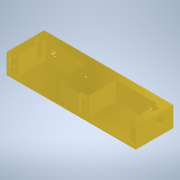
# Autodesk Inventor part: Part4
Saved by Autodesk Inventor 2022 (Build 260153000, 153)
## iProperties
Created: 2021-06-22
Part Number: Part4
Material: Generic
Document SubType Name: Modeling
Designer: Prajwal Patil
Density: 1 g/cm^3
Appearance: Diamond Plate
Author: Prajwal Patil
Autodesk Inventor part; units mm, degrees
ref_plane "YZ Plane" through (0, 0, 0) normal (1, 0, 0) x (0, 1, 0)
ref_plane "XZ Plane" through (0, 0, 0) normal (0, 1, 0) x (-1, 0, 0)
ref_plane "XY Plane" through (0, 0, 0) normal (0, 0, 1) x (1, 0, 0)
sketch "Sketch2" plane through (0, 0, 0) normal (0, 1, 0) x (-1, 0, 0)
  line L0 (77.2994, 22.4824) -> (-85.2606, 22.4824)
  line L1 (-85.2606, 22.4824) -> (-85.2606, -24.5076)
  line L2 (-85.2606, -24.5076) -> (77.2994, -24.5076)
  line L3 (77.2994, -24.5076) -> (77.2994, 22.4824)
  point P0 (0, 0)
  dimension "d0" = 162.56
  dimension "d1" = 46.99
  constraints: 8 end point, 2 parallel, 1 horizontal, 1 perpendicular
  measures "d0" distance of L2.end L1.end
  measures "d1" distance of L1.end L0.end
extrude "Extrusion1" add sketch "Sketch2" along normal blind 25.4
sketch "Sketch3" plane through (0, 25.4, 0) normal (0, 1, 0) x (1, 0, 0)
  point P0 (0, 0)
sketch "Sketch4" plane through (0, 25.4, 0) normal (0, 1, 0) x (1, 0, 0)
  line L0 (85.2606, -22.4824) -> (85.2606, 24.5076) projected
  line L1 (74.5926, -22.4824) -> (74.5926, 15.6176)
  line L2 (74.5926, 15.6176) -> (22.2686, 15.6176)
  line L3 (22.2686, 15.6176) -> (22.2686, -22.4824)
  line L4 (-14.3074, -22.4824) -> (-14.3074, 15.6176)
  line L5 (-14.3074, 15.6176) -> (-66.6314, 15.6176)
  line L6 (-66.6314, 15.6176) -> (-66.6314, -22.4824)
  line L7 (-66.6314, -22.4824) -> (-14.3074, -22.4824)
  line L8 (22.2686, -22.4824) -> (74.5926, -22.4824)
  point P0 (0, 0)
  dimension "d4" = 10.668
  dimension "d5" = 38.1
  dimension "d6" = 52.324
  dimension "d7" = 36.576
  dimension "d8" = 52.324
  constraints: 16 end point, 3 perpendicular, 1 collinear
  measures "d4" distance of L0.start L1.start
  measures "d5" distance of L1.start L1.end
  measures "d6" distance of L1.end L2.end
  measures "d7" distance of L3.end L4.start
  measures "d8" distance of L4.end L5.end
extrude "Extrusion2" cut sketch "Sketch4" against normal blind 23.495
sketch "Sketch5" plane through (0, 25.4, 0) normal (0, 1, 0) x (1, 0, 0)
  line L0 (74.5926, -22.4824) -> (22.2686, -22.4824) projected
  line L1 (22.2686, -22.4824) -> (13.5564, -22.4824)
  line L2 (13.5564, -22.4824) -> (13.5564, -18.6724)
  line L3 (13.5564, -18.6724) -> (22.2686, -18.6724)
  line L4 (22.2686, -18.6724) -> (22.2686, -22.4824)
  line L5 (-14.3074, -22.4824) -> (22.2686, -22.4824) projected
  line L6 (-14.3074, -22.4824) -> (-5.5952, -22.4824)
  line L7 (-5.5952, -22.4824) -> (-5.5952, -18.6724)
  line L8 (-5.5952, -18.6724) -> (-14.3074, -18.6724)
  line L9 (-14.3074, -18.6724) -> (-14.3074, -22.4824)
  line L10 (74.5926, -22.4824) -> (85.2606, -22.4824) projected
  line L11 (74.5926, -22.4824) -> (83.3048, -22.4824)
  line L12 (83.3048, -22.4824) -> (83.3048, -18.6724)
  line L13 (83.3048, -18.6724) -> (74.5926, -18.6724)
  line L14 (74.5926, -18.6724) -> (74.5926, -22.4824)
  line L15 (-66.6314, -22.4824) -> (-66.6314, 15.6176) projected
  line L16 (-66.6314, -22.4824) -> (-75.3436, -22.4824)
  line L17 (-75.3436, -22.4824) -> (-75.3436, -18.6724)
  line L18 (-75.3436, -18.6724) -> (-66.6314, -18.6724)
  line L19 (-66.6314, -18.6724) -> (-66.6314, -22.4824)
  point P0 (0, 0)
  point P1 (-77.2994, -22.4824)
  dimension "d11" = 8.7122
  dimension "d12" = 3.81
  dimension "d13" = 8.7122
  dimension "d14" = 3.81
  dimension "d18" = 8.7122
  dimension "d19" = 8.7122
  dimension "d20" = 3.81
  constraints: 32 end point, 8 parallel, 4 horizontal, 4 perpendicular
  measures "d11" distance of L2.end L3.end
  measures "d12" distance of L1.end L2.end
  measures "d13" distance of L8.end L7.end
  measures "d14" distance of L7.end L6.end
  measures "d18" distance of L13.end L12.end
  measures "d19" distance of L17.end L18.end
  measures "d20" distance of L16.end L17.end
extrude "Extrusion3" cut sketch "Sketch5" against normal blind 22.5552
sketch "Sketch6" plane through (0, 25.4, 0) normal (0, 1, 0) x (1, 0, 0)
  line L0 (74.5926, 12.4426) -> (79.7234, 12.4426)
  line L1 (79.7234, 12.4426) -> (79.7234, 4.8226)
  line L2 (79.7234, 4.8226) -> (74.5926, 4.8226)
  line L3 (74.5926, 12.4426) -> (74.5926, 4.8226)
  line L4 (-66.6314, 12.4426) -> (-71.7622, 12.4426)
  line L5 (-71.7622, 12.4426) -> (-71.7622, 4.8226)
  line L6 (-71.7622, 4.8226) -> (-66.6314, 4.8226)
  line L7 (-66.6314, 4.8226) -> (-66.6314, 12.4426)
  point P0 (0, 0)
  point P1 (74.5926, 15.6176)
  point P2 (-66.6314, 15.6176)
  dimension "d23" = 3.175
  dimension "d24" = 5.1308
  dimension "d25" = 7.62
  dimension "d26" = 3.175
  dimension "d27" = 5.1308
  constraints: 16 end point, 3 perpendicular, 2 horizontal, 1 vertical
  measures "d23" distance of point (74.593, 15.618) L0.start
  measures "d24" distance of L0.start L0.end
  measures "d25" distance of L0.end L1.end
  measures "d26" distance of point (-66.631, 15.618) L4.start
  measures "d27" distance of L4.start L4.end
extrude "Extrusion4" cut sketch "Sketch6" against normal blind 15.875
sketch "Sketch7" plane through (85.2606, 0, 22.4824) normal (1, 0, 0) x (0, 0, -1)
  point P0 (22.4824, 0)
sketch "Sketch8" plane through (85.2606, 0, 22.4824) normal (1, 0, 0) x (0, 0, -1)
  line L0 (27.305, 9.525) -> (34.925, 9.525) projected
  line L1 (27.305, 25.4) -> (27.305, 9.525) projected
  line L2 (34.925, 9.525) -> (27.305, 9.525)
  line L3 (27.305, 9.525) -> (27.305, 20.955)
  line L4 (27.305, 20.955) -> (34.925, 20.955)
  line L5 (38.1, 25.4) -> (38.1, 1.905) projected
  line L6 (34.925, 20.955) -> (34.925, 9.525)
  point P0 (22.4824, 0)
  point P1 (46.99, 0)
  dimension "d32" = 11.43
  constraints: 8 end point, 1 perpendicular, 1 point on line
  measures "d32" distance of L0.start L3.end
extrude "Extrusion5" cut sketch "Sketch8" against normal blind 10.3124
sketch "Sketch10" plane through (-77.2994, 0, -24.5076) normal (-1, 0, 0) x (0, 0, 1)
  line L0 (19.685, 20.955) -> (12.065, 20.955) projected
  line L1 (19.685, 9.525) -> (19.685, 20.955) projected
  line L2 (12.065, 20.955) -> (19.685, 20.955)
  line L3 (19.685, 20.955) -> (19.685, 9.525)
  line L4 (19.685, 9.525) -> (12.065, 9.525)
  line L5 (12.065, 9.525) -> (12.065, 20.955)
  point P0 (24.5076, 0)
  constraints: 8 end point, 2 parallel, 1 horizontal, 1 perpendicular
extrude "Extrusion6" cut sketch "Sketch10" against normal blind 10.3124
sketch "Sketch12" plane through (74.5926, 25.4, 18.6724) normal (0, 0, 1) x (1, 0, 0)
  line L0 (8.7122, -22.5552) -> (4.9022, -22.5552)
  line L1 (-61.0362, 0) -> (-61.0362, -22.5552) projected
  line L2 (-61.0362, -22.5552) -> (-57.2262, -22.5552)
  line L3 (-61.0362, -22.5552) -> (-52.324, -22.5552) projected
  line L4 (8.7122, -22.5552) -> (0, -22.5552) projected
  line L5 (8.7122, -22.5552) -> (4.9022, -22.5552)
  line L6 (10.668, -15.875) -> (0, -15.875) projected
  line L7 (4.9022, -22.5552) -> (12.5222, -22.5552) construction
  circle A0 centre (4.9022, -14.9352) radius 1.27
  circle A1 centre (4.9022, -4.1402) radius 1.27
  circle A2 centre (-57.2262, -4.1402) radius 1.27
  circle A3 centre (-57.2262, -14.9352) radius 1.27
  line L8 (-80.1878, -22.5552) -> (-83.9978, -22.5552)
  line L9 (-80.1878, -22.5552) -> (-88.9, -22.5552) projected
  circle A4 centre (-83.9978, -4.1402) radius 1.27
  circle A5 centre (-83.9978, -14.9352) radius 1.27
  line L10 (-141.224, -22.5552) -> (-149.9362, -22.5552) projected
  line L11 (-149.9362, -22.5552) -> (-146.1262, -22.5552)
  line L12 (-146.1262, -14.9352) -> (-135.3312, -14.9352) construction
  circle A6 centre (-146.1262, -14.9352) radius 1.27
  circle A7 centre (-146.1262, -4.1402) radius 1.27
  point P0 (-74.5926, -25.4)
  dimension "d48" = 3.81
  dimension "d55" = 2.54
  dimension "d56" = 2.54
  dimension "d57" = 3.81
  dimension "d58" = 2.54
  dimension "d59" = 2.54
  dimension "d60" = 3.81
  dimension "d64" = 2.54
  dimension "d65" = 2.54
  constraints: 14 end point, 8 centre point, 3 point on line, 2 horizontal, 1 coincident, 1 collinear
  measures "d48" distance of L1.end L2.end
  measures "d55" diameter of A0
  measures "d56" diameter of A1
  measures "d57" distance of L8.start L8.end
  measures "d58" diameter of A4
  measures "d59" diameter of A5
  measures "d60" distance of L10.end L11.end
  measures "d64" diameter of A6
  measures "d65" diameter of A7
extrude "Extrusion7" cut sketch "Sketch12" against normal blind 10.16
sketch "Sketch13" plane through (22.2686, 25.4, -15.6176) normal (0, 0, 1) x (1, 0, 0)
  line L0 (52.324, -23.495) -> (0, -23.495) projected
  line L1 (52.324, -23.495) -> (42.164, -23.495)
  circle A0 centre (42.164, -10.16) radius 3.81
  line L2 (-88.9, -23.495) -> (-36.576, -23.495) projected
  line L3 (-88.9, -23.495) -> (-78.74, -23.495)
  line L4 (62.992, -25.4) -> (-99.568, -25.4) projected
  line L5 (-88.9, -23.495) -> (-78.74, -23.495) construction
  circle A1 centre (-78.74, -10.16) radius 3.81
  point P0 (-22.2686, -25.4)
  dimension "d68" = 10.16
  dimension "d70" = 7.62
  dimension "d71" = 10.16
  dimension "d72" = 0
  dimension "d73" = 7.62
  constraints: 6 end point, 2 centre point, 1 collinear, 1 horizontal, 1 parallel, 1 point on line
  measures "d68" distance of L0.start L1.end
  measures "d70" diameter of A0
  measures "d71" distance of L2.start L3.end
  measures "d72" distance between parallel lines of L3 L5
  measures "d73" diameter of A1
extrude "Extrusion8" cut sketch "Sketch13" against normal blind 8.89
sketch "Sketch14" plane through (0, 0, 0) normal (0, -1, 0) x (1, 0, 0)
  line L0 (-74.5451, 20.5131) -> (78.1896, 20.5131) construction
  line L1 (78.1896, 20.5131) -> (78.1896, -20.8075) construction
  line L2 (78.1896, -20.8075) -> (-74.5451, -20.8075) construction
  line L3 (-74.5451, -20.8075) -> (-74.5451, 20.5131) construction
  spline S0 degree 2 poles (-33.4111, 7.8193) (-33.4111, 6.4937) (-34.4197, 4.4621) (-35.2554, 3.7993) knots 0 0 0 1 2 2 2
  spline S1 degree 2 poles (-35.2554, 3.7993) (-36.264, 3.0213) (-38.5549, 2.3585) (-40.3704, 2.3585) knots 0 0 0 1 2 2 2
  line L4 (-40.3704, 2.3585) -> (-45.471, 2.3585)
  line L5 (-45.471, 2.3585) -> (-45.471, 20.1385)
  line L6 (-45.471, 20.1385) -> (-40.7594, 20.1385)
  spline S2 degree 2 poles (-40.7594, 20.1385) (-38.8575, 20.1385) (-36.9556, 19.8935) (-36.0911, 19.4181) knots 0 0 0 1 2 2 2
  spline S3 degree 2 poles (-36.0911, 19.4181) (-35.1257, 18.9138) (-34.2468, 17.2568) (-34.2468, 16.1329) knots 0 0 0 1 2 2 2
  spline S4 degree 2 poles (-34.2468, 16.1329) (-34.2468, 14.8794) (-35.5724, 12.891) (-36.7394, 12.3291) knots 0 0 0 1 2 2 2
  line L7 (-36.7394, 12.3291) -> (-36.7394, 12.2427)
  spline S5 degree 2 poles (-36.7394, 12.2427) (-35.1545, 11.8104) (-33.4111, 9.5195) (-33.4111, 7.8193) knots 0 0 0 1 2 2 2
  spline S6 degree 2 poles (-35.8749, 7.7184) (-35.8749, 8.727) (-36.4513, 10.0238) (-37.3158, 10.4848) knots 0 0 0 1 2 2 2
  spline S7 degree 2 poles (-37.3158, 10.4848) (-37.8777, 10.773) (-39.2033, 10.9459) (-40.428, 10.9459) knots 0 0 0 1 2 2 2
  line L8 (-40.428, 10.9459) -> (-43.108, 10.9459)
  line L9 (-43.108, 10.9459) -> (-43.108, 4.3757)
  line L10 (-43.108, 4.3757) -> (-41.1917, 4.3757)
  spline S8 degree 2 poles (-41.1917, 4.3757) (-39.6355, 4.3757) (-37.8489, 4.6638) (-37.1573, 5.1249) knots 0 0 0 1 2 2 2
  spline S9 degree 2 poles (-37.1573, 5.1249) (-36.4945, 5.6004) (-35.8749, 6.7819) (-35.8749, 7.7184) knots 0 0 0 1 2 2 2
  spline S10 degree 2 poles (-36.7106, 15.8015) (-36.7106, 16.4355) (-37.1429, 17.3865) (-37.6184, 17.6602) knots 0 0 0 1 2 2 2
  spline S11 degree 2 poles (-37.6184, 17.6602) (-38.1947, 17.9772) (-39.5923, 18.1213) (-40.8459, 18.1213) knots 0 0 0 1 2 2 2
  line L11 (-40.8459, 18.1213) -> (-43.108, 18.1213)
  line L12 (-43.108, 18.1213) -> (-43.108, 12.9199)
  line L13 (-43.108, 12.9199) -> (-40.428, 12.9199)
  spline S12 degree 2 poles (-40.428, 12.9199) (-39.3186, 12.9199) (-38.2667, 13.1504) (-37.7048, 13.5106) knots 0 0 0 1 2 2 2
  spline S13 degree 2 poles (-37.7048, 13.5106) (-37.1573, 13.8564) (-36.7106, 14.9658) (-36.7106, 15.8015) knots 0 0 0 1 2 2 2
  spline S14 degree 2 poles (-18.484, 18.1069) (-17.4754, 16.9254) (-16.3515, 13.4674) (-16.3515, 11.2485) knots 0 0 0 1 2 2 2
  spline S15 degree 2 poles (-16.3515, 11.2485) (-16.3515, 9.0872) (-17.4466, 5.586) (-18.484, 4.4045) knots 0 0 0 1 2 2 2
  spline S16 degree 2 poles (-18.484, 4.4045) (-19.579, 3.1653) (-22.4751, 1.9839) (-24.2185, 1.9839) knots 0 0 0 1 2 2 2
  spline S17 degree 2 poles (-24.2185, 1.9839) (-26.0196, 1.9839) (-28.9013, 3.2086) (-29.9531, 4.4045) knots 0 0 0 1 2 2 2
  spline S18 degree 2 poles (-29.9531, 4.4045) (-30.9761, 5.586) (-32.0711, 9.0584) (-32.0711, 11.2485) knots 0 0 0 1 2 2 2
  spline S19 degree 2 poles (-32.0711, 11.2485) (-32.0711, 13.4818) (-30.9617, 16.8822) (-29.9387, 18.1069) knots 0 0 0 1 2 2 2
  spline S20 degree 2 poles (-29.9387, 18.1069) (-28.9013, 19.2884) (-26.0052, 20.5131) (-24.2185, 20.5131) knots 0 0 0 1 2 2 2
  spline S21 degree 2 poles (-24.2185, 20.5131) (-22.4031, 20.5131) (-19.4926, 19.2452) (-18.484, 18.1069) knots 0 0 0 1 2 2 2
  spline S22 degree 2 poles (-18.8154, 11.2485) (-18.8154, 13.0063) (-19.579, 15.7295) (-20.2706, 16.6228) knots 0 0 0 1 2 2 2
  spline S23 degree 2 poles (-20.2706, 16.6228) (-20.9766, 17.545) (-22.965, 18.4671) (-24.2041, 18.4671) knots 0 0 0 1 2 2 2
  spline S24 degree 2 poles (-24.2041, 18.4671) (-25.4865, 18.4671) (-27.4172, 17.5738) (-28.152, 16.6228) knots 0 0 0 1 2 2 2
  spline S25 degree 2 poles (-28.152, 16.6228) (-28.858, 15.7151) (-29.6073, 12.9775) (-29.6073, 11.2485) knots 0 0 0 1 2 2 2
  spline S26 degree 2 poles (-29.6073, 11.2485) (-29.6073, 7.7472) (-26.668, 4.0299) (-24.2041, 4.0299) knots 0 0 0 1 2 2 2
  spline S27 degree 2 poles (-24.2041, 4.0299) (-21.7403, 4.0299) (-18.8154, 7.7472) (-18.8154, 11.2485) knots 0 0 0 1 2 2 2
  line L14 (-9.6084, 2.3585) -> (-9.6084, 18.0348)
  line L15 (-9.6084, 18.0348) -> (-15.5735, 18.0348)
  line L16 (-15.5735, 18.0348) -> (-15.5735, 20.1385)
  line L17 (-15.5735, 20.1385) -> (-1.2803, 20.1385)
  line L18 (-1.2803, 20.1385) -> (-1.2803, 18.0348)
  line L19 (-1.2803, 18.0348) -> (-7.2454, 18.0348)
  line L20 (-7.2454, 18.0348) -> (-7.2454, 2.3585)
  line L21 (-7.2454, 2.3585) -> (-9.6084, 2.3585)
  line L22 (6.5291, 9.0584) -> (-0.1997, 9.0584)
  line L23 (-0.1997, 9.0584) -> (-0.1997, 11.2197)
  line L24 (-0.1997, 11.2197) -> (6.5291, 11.2197)
  line L25 (6.5291, 11.2197) -> (6.5291, 9.0584)
  line L26 (18.9635, 2.3585) -> (10.2897, 2.3585)
  line L27 (10.2897, 2.3585) -> (10.2897, 4.1739)
  line L28 (10.2897, 4.1739) -> (13.5171, 4.1739)
  line L29 (13.5171, 4.1739) -> (13.5171, 16.0897)
  line L30 (13.5171, 16.0897) -> (10.2897, 16.0897)
  line L31 (10.2897, 16.0897) -> (10.2897, 17.7179)
  spline S28 degree 2 poles (10.2897, 17.7179) (12.1195, 17.7179) (13.8485, 18.7553) (13.9638, 20.1961) knots 0 0 0 1 2 2 2
  line L32 (13.9638, 20.1961) -> (15.8081, 20.1961)
  line L33 (15.8081, 20.1961) -> (15.8081, 4.1739)
  line L34 (15.8081, 4.1739) -> (18.9635, 4.1739)
  line L35 (18.9635, 4.1739) -> (18.9635, 2.3585)
  spline S29 degree 2 poles (33.4728, 8.1218) (33.4728, 6.753) (32.5651, 4.4333) (31.8014, 3.6552) knots 0 0 0 1 2 2 2
  spline S30 degree 2 poles (31.8014, 3.6552) (31.009, 2.834) (29.0206, 1.9839) (27.8247, 1.9839) knots 0 0 0 1 2 2 2
  spline S31 degree 2 poles (27.8247, 1.9839) (26.6288, 1.9839) (24.6549, 2.7907) (23.9056, 3.5976) knots 0 0 0 1 2 2 2
  spline S32 degree 2 poles (23.9056, 3.5976) (22.9835, 4.563) (21.9461, 7.8049) (21.9461, 10.1678) knots 0 0 0 1 2 2 2
  spline S33 degree 2 poles (21.9461, 10.1678) (21.9461, 12.4876) (22.897, 16.2194) (23.8912, 17.6026) knots 0 0 0 1 2 2 2
  spline S34 degree 2 poles (23.8912, 17.6026) (24.8566, 18.957) (27.9112, 20.4699) (29.9139, 20.4699) knots 0 0 0 1 2 2 2
  spline S35 degree 2 poles (29.9139, 20.4699) (30.5047, 20.4699) (31.5421, 20.3546) (31.9311, 20.2249) knots 0 0 0 1 2 2 2
  line L36 (31.9311, 20.2249) -> (31.9311, 17.934)
  line L37 (31.9311, 17.934) -> (31.8303, 17.934)
  spline S36 degree 2 poles (31.8303, 17.934) (31.4989, 18.1069) (30.2886, 18.4095) (29.597, 18.4095) knots 0 0 0 1 2 2 2
  spline S37 degree 2 poles (29.597, 18.4095) (27.3781, 18.4095) (24.6549, 15.4125) (24.3955, 12.4732) knots 0 0 0 1 2 2 2
  spline S38 degree 2 poles (24.3955, 12.4732) (25.2456, 13.0639) (27.0323, 13.7123) (28.0985, 13.7123) knots 0 0 0 1 2 2 2
  spline S39 degree 2 poles (28.0985, 13.7123) (29.1359, 13.7123) (30.692, 13.2945) (31.5421, 12.6605) knots 0 0 0 1 2 2 2
  spline S40 degree 2 poles (31.5421, 12.6605) (32.5219, 11.9257) (33.4728, 9.6491) (33.4728, 8.1218) knots 0 0 0 1 2 2 2
  spline S41 degree 2 poles (31.0522, 8.021) (31.0522, 9.116) (30.4759, 10.6001) (29.8419, 11.1188) knots 0 0 0 1 2 2 2
  spline S42 degree 2 poles (29.8419, 11.1188) (29.3664, 11.4934) (28.1849, 11.7384) (27.5654, 11.7384) knots 0 0 0 1 2 2 2
  spline S43 degree 2 poles (27.5654, 11.7384) (26.7297, 11.7384) (25.1592, 11.2341) (24.3955, 10.7586) knots 0 0 0 1 2 2 2
  spline S44 degree 2 poles (24.3955, 10.7586) (24.3811, 10.4992) (24.3523, 10.0093) (24.3523, 9.6347) knots 0 0 0 1 2 2 2
  spline S45 degree 2 poles (24.3523, 9.6347) (24.3523, 7.7905) (25.0727, 5.5283) (25.6202, 4.9376) knots 0 0 0 1 2 2 2
  spline S46 degree 2 poles (25.6202, 4.9376) (26.1245, 4.3757) (27.2196, 3.929) (27.8391, 3.929) knots 0 0 0 1 2 2 2
  spline S47 degree 2 poles (27.8391, 3.929) (29.28, 3.929) (31.0522, 5.975) (31.0522, 8.021) knots 0 0 0 1 2 2 2
  spline S48 degree 2 poles (-38.1227, -15.5926) (-38.1227, -17.9289) (-40.3868, -20.7797) (-42.0953, -20.7797) knots 0 0 0 1 2 2 2
  spline S49 degree 2 poles (-42.0953, -20.7797) (-42.8671, -20.7797) (-43.9684, -20.3989) (-44.5035, -20.0695) knots 0 0 0 1 2 2 2
  line L38 (-44.5035, -20.0695) -> (-44.6064, -20.5121)
  line L39 (-44.6064, -20.5121) -> (-46.109, -20.5121)
  line L40 (-46.109, -20.5121) -> (-46.109, -7.246)
  line L41 (-46.109, -7.246) -> (-44.5035, -7.246)
  line L42 (-44.5035, -7.246) -> (-44.5035, -11.9802)
  spline S50 degree 2 poles (-44.5035, -11.9802) (-43.8963, -11.4348) (-42.4864, -10.7144) (-41.591, -10.7144) knots 0 0 0 1 2 2 2
  spline S51 degree 2 poles (-41.591, -10.7144) (-39.9752, -10.7144) (-38.1227, -13.2976) (-38.1227, -15.5926) knots 0 0 0 1 2 2 2
  spline S52 degree 2 poles (-39.7796, -15.7161) (-39.7796, -14.0077) (-40.8191, -12.2375) (-41.9718, -12.2375) knots 0 0 0 1 2 2 2
  spline S53 degree 2 poles (-41.9718, -12.2375) (-42.6201, -12.2375) (-43.9581, -12.855) (-44.5035, -13.3285) knots 0 0 0 1 2 2 2
  line L43 (-44.5035, -13.3285) -> (-44.5035, -18.7934)
  spline S54 degree 2 poles (-44.5035, -18.7934) (-43.8963, -19.0918) (-42.9598, -19.3388) (-42.404, -19.3388) knots 0 0 0 1 2 2 2
  spline S55 degree 2 poles (-42.404, -19.3388) (-41.1793, -19.3388) (-39.7796, -17.5995) (-39.7796, -15.7161) knots 0 0 0 1 2 2 2
  line L44 (-28.9733, -10.9819) -> (-34.0986, -24.0216)
  line L45 (-34.0986, -24.0216) -> (-35.8173, -24.0216)
  line L46 (-35.8173, -24.0216) -> (-34.1089, -20.049)
  line L47 (-34.1089, -20.049) -> (-37.5669, -10.9819)
  line L48 (-37.5669, -10.9819) -> (-35.8379, -10.9819)
  line L49 (-35.8379, -10.9819) -> (-33.2341, -18.0421)
  line L50 (-33.2341, -18.0421) -> (-30.6406, -10.9819)
  line L51 (-30.6406, -10.9819) -> (-28.9733, -10.9819)
  line L52 (-19.2167, -20.5121) -> (-19.2167, -9.3147)
  line L53 (-19.2167, -9.3147) -> (-23.4775, -9.3147)
  line L54 (-23.4775, -9.3147) -> (-23.4775, -7.8121)
  line L55 (-23.4775, -7.8121) -> (-13.2681, -7.8121)
  line L56 (-13.2681, -7.8121) -> (-13.2681, -9.3147)
  line L57 (-13.2681, -9.3147) -> (-17.5289, -9.3147)
  line L58 (-17.5289, -9.3147) -> (-17.5289, -20.5121)
  line L59 (-17.5289, -20.5121) -> (-19.2167, -20.5121)
  spline S56 degree 2 poles (-7.9679, -20.7282) (-10.2526, -20.7282) (-12.7638, -18.1656) (-12.7638, -15.7985) knots 0 0 0 1 2 2 2
  spline S57 degree 2 poles (-12.7638, -15.7985) (-12.7638, -13.4725) (-10.3247, -10.7144) (-8.359, -10.7144) knots 0 0 0 1 2 2 2
  spline S58 degree 2 poles (-8.359, -10.7144) (-7.4739, -10.7144) (-6.1051, -11.2289) (-5.6008, -11.7744) knots 0 0 0 1 2 2 2
  spline S59 degree 2 poles (-5.6008, -11.7744) (-5.0862, -12.3199) (-4.5407, -13.8945) (-4.5407, -15.0369) knots 0 0 0 1 2 2 2
  line L60 (-4.5407, -15.0369) -> (-4.5407, -15.9117)
  line L61 (-4.5407, -15.9117) -> (-11.1377, -15.9117)
  spline S60 degree 2 poles (-11.1377, -15.9117) (-11.1377, -17.5686) (-9.4705, -19.3285) (-7.9885, -19.3285) knots 0 0 0 1 2 2 2
  spline S61 degree 2 poles (-7.9885, -19.3285) (-7.4636, -19.3285) (-6.4447, -19.0918) (-6.033, -18.9066) knots 0 0 0 1 2 2 2
  spline S62 degree 2 poles (-6.033, -18.9066) (-5.6008, -18.7007) (-5.0039, -18.3405) (-4.8083, -18.1759) knots 0 0 0 1 2 2 2
  line L62 (-4.8083, -18.1759) -> (-4.7157, -18.1759)
  line L63 (-4.7157, -18.1759) -> (-4.7157, -19.9255)
  spline S63 degree 2 poles (-4.7157, -19.9255) (-4.9936, -20.0387) (-5.8375, -20.368) (-6.1668, -20.4606) knots 0 0 0 1 2 2 2
  spline S64 degree 2 poles (-6.1668, -20.4606) (-6.63, -20.5944) (-7.3915, -20.7282) (-7.9679, -20.7282) knots 0 0 0 1 2 2 2
  spline S65 degree 2 poles (-6.1051, -14.687) (-6.1257, -14.0386) (-6.3932, -13.0917) (-6.6505, -12.7727) knots 0 0 0 1 2 2 2
  spline S66 degree 2 poles (-6.6505, -12.7727) (-6.9284, -12.4125) (-7.8032, -12.0317) (-8.4516, -12.0317) knots 0 0 0 1 2 2 2
  spline S67 degree 2 poles (-8.4516, -12.0317) (-9.0897, -12.0317) (-9.9851, -12.4125) (-10.3556, -12.783) knots 0 0 0 1 2 2 2
  spline S68 degree 2 poles (-10.3556, -12.783) (-10.7158, -13.1638) (-11.0863, -14.0798) (-11.1377, -14.687) knots 0 0 0 1 2 2 2
  line L64 (-11.1377, -14.687) -> (-6.1051, -14.687)
  spline S69 degree 2 poles (2.3959, -19.5035) (2.2004, -19.6476) (1.5417, -20.1622) (1.2329, -20.3165) knots 0 0 0 1 2 2 2
  spline S70 degree 2 poles (1.2329, -20.3165) (0.811, -20.543) (0.0185, -20.7797) (-0.7019, -20.7797) knots 0 0 0 1 2 2 2
  spline S71 degree 2 poles (-0.7019, -20.7797) (-1.2885, -20.7797) (-2.3486, -20.3371) (-2.75, -19.9357) knots 0 0 0 1 2 2 2
  spline S72 degree 2 poles (-2.75, -19.9357) (-3.1308, -19.5447) (-3.5939, -18.392) (-3.5939, -17.7539) knots 0 0 0 1 2 2 2
  spline S73 degree 2 poles (-3.5939, -17.7539) (-3.5939, -16.7659) (-2.7603, -15.3662) (-1.8546, -14.9648) knots 0 0 0 1 2 2 2
  spline S74 degree 2 poles (-1.8546, -14.9648) (-1.0518, -14.5943) (1.13, -14.3165) (2.3959, -14.2444) knots 0 0 0 1 2 2 2
  line L65 (2.3959, -14.2444) -> (2.3959, -13.9357)
  spline S75 degree 2 poles (2.3959, -13.9357) (2.3959, -13.3799) (2.0563, -12.6904) (1.7475, -12.4948) knots 0 0 0 1 2 2 2
  spline S76 degree 2 poles (1.7475, -12.4948) (1.4388, -12.2993) (0.5537, -12.1758) (0.0803, -12.1758) knots 0 0 0 1 2 2 2
  spline S77 degree 2 poles (0.0803, -12.1758) (-0.4755, -12.1758) (-1.9781, -12.5051) (-2.7294, -12.8242) knots 0 0 0 1 2 2 2
  line L66 (-2.7294, -12.8242) -> (-2.822, -12.8242)
  line L67 (-2.822, -12.8242) -> (-2.822, -11.1878)
  spline S78 degree 2 poles (-2.822, -11.1878) (-2.3795, -11.0643) (-0.7225, -10.7555) (0.0906, -10.7555) knots 0 0 0 1 2 2 2
  spline S79 degree 2 poles (0.0906, -10.7555) (1.0786, -10.7555) (2.4268, -11.0643) (2.9619, -11.4657) knots 0 0 0 1 2 2 2
  spline S80 degree 2 poles (2.9619, -11.4657) (3.4868, -11.8567) (4.0014, -13.102) (4.0014, -13.9974) knots 0 0 0 1 2 2 2
  line L68 (4.0014, -13.9974) -> (4.0014, -20.5121)
  line L69 (4.0014, -20.5121) -> (2.3959, -20.5121)
  line L70 (2.3959, -20.5121) -> (2.3959, -19.5035)
  line L71 (2.3959, -18.1656) -> (2.3959, -15.5206)
  spline S81 degree 2 poles (2.3959, -15.5206) (1.8196, -15.5721) (0.0803, -15.747) (-0.4652, -15.9117) knots 0 0 0 1 2 2 2
  spline S82 degree 2 poles (-0.4652, -15.9117) (-1.1033, -16.1072) (-1.9369, -16.9203) (-1.9369, -17.6407) knots 0 0 0 1 2 2 2
  spline S83 degree 2 poles (-1.9369, -17.6407) (-1.9369, -18.464) (-1.0107, -19.2977) (-0.1256, -19.2977) knots 0 0 0 1 2 2 2
  spline S84 degree 2 poles (-0.1256, -19.2977) (0.6257, -19.2977) (1.8607, -18.6493) (2.3959, -18.1656) knots 0 0 0 1 2 2 2
  line L72 (17.0616, -20.5121) -> (17.0616, -14.9957)
  spline S85 degree 2 poles (17.0616, -14.9957) (17.0616, -14.337) (16.9587, -13.2152) (16.794, -12.9065) knots 0 0 0 1 2 2 2
  spline S86 degree 2 poles (16.794, -12.9065) (16.6294, -12.5669) (16.0016, -12.2375) (15.4561, -12.2375) knots 0 0 0 1 2 2 2
  spline S87 degree 2 poles (15.4561, -12.2375) (14.9621, -12.2375) (13.83, -12.8447) (13.2331, -13.4211) knots 0 0 0 1 2 2 2
  spline S88 degree 2 poles (13.2331, -13.4211) (13.2434, -13.5652) (13.264, -13.9665) (13.264, -14.2341) knots 0 0 0 1 2 2 2
  line L73 (13.264, -14.2341) -> (13.264, -20.5121)
  line L74 (13.264, -20.5121) -> (11.6585, -20.5121)
  line L75 (11.6585, -20.5121) -> (11.6585, -14.9957)
  spline S89 degree 2 poles (11.6585, -14.9957) (11.6585, -14.337) (11.5555, -13.2152) (11.3909, -12.9065) knots 0 0 0 1 2 2 2
  spline S90 degree 2 poles (11.3909, -12.9065) (11.2262, -12.5669) (10.5984, -12.2375) (10.053, -12.2375) knots 0 0 0 1 2 2 2
  spline S91 degree 2 poles (10.053, -12.2375) (9.5384, -12.2375) (8.396, -12.8859) (7.8608, -13.3902) knots 0 0 0 1 2 2 2
  line L76 (7.8608, -13.3902) -> (7.8608, -20.5121)
  line L77 (7.8608, -20.5121) -> (6.2553, -20.5121)
  line L78 (6.2553, -20.5121) -> (6.2553, -10.9819)
  line L79 (6.2553, -10.9819) -> (7.8608, -10.9819)
  line L80 (7.8608, -10.9819) -> (7.8608, -12.0317)
  spline S92 degree 2 poles (7.8608, -12.0317) (8.4886, -11.4039) (9.7236, -10.7144) (10.4646, -10.7144) knots 0 0 0 1 2 2 2
  spline S93 degree 2 poles (10.4646, -10.7144) (11.3085, -10.7144) (12.6156, -11.4862) (12.9552, -12.361) knots 0 0 0 1 2 2 2
  spline S94 degree 2 poles (12.9552, -12.361) (13.6859, -11.548) (15.065, -10.7144) (15.8678, -10.7144) knots 0 0 0 1 2 2 2
  spline S95 degree 2 poles (15.8678, -10.7144) (16.4853, -10.7144) (17.4939, -11.0951) (17.8644, -11.5274) knots 0 0 0 1 2 2 2
  spline S96 degree 2 poles (17.8644, -11.5274) (18.2452, -11.9597) (18.6671, -13.2564) (18.6671, -14.2341) knots 0 0 0 1 2 2 2
  line L81 (18.6671, -14.2341) -> (18.6671, -20.5121)
  line L82 (18.6671, -20.5121) -> (17.0616, -20.5121)
  line L83 (33.3329, -20.5121) -> (27.1372, -20.5121)
  line L84 (27.1372, -20.5121) -> (27.1372, -19.2153)
  line L85 (27.1372, -19.2153) -> (29.4426, -19.2153)
  line L86 (29.4426, -19.2153) -> (29.4426, -10.7041)
  line L87 (29.4426, -10.7041) -> (27.1372, -10.7041)
  line L88 (27.1372, -10.7041) -> (27.1372, -9.5411)
  spline S97 degree 2 poles (27.1372, -9.5411) (28.4443, -9.5411) (29.6793, -8.8001) (29.7616, -7.7709) knots 0 0 0 1 2 2 2
  line L89 (29.7616, -7.7709) -> (31.079, -7.7709)
  line L90 (31.079, -7.7709) -> (31.079, -19.2153)
  line L91 (31.079, -19.2153) -> (33.3329, -19.2153)
  line L92 (33.3329, -19.2153) -> (33.3329, -20.5121)
  spline S98 degree 2 poles (43.6966, -16.3954) (43.6966, -17.3731) (43.0482, -19.0301) (42.5028, -19.5858) knots 0 0 0 1 2 2 2
  spline S99 degree 2 poles (42.5028, -19.5858) (41.9367, -20.1725) (40.5165, -20.7797) (39.6623, -20.7797) knots 0 0 0 1 2 2 2
  spline S100 degree 2 poles (39.6623, -20.7797) (38.8081, -20.7797) (37.3981, -20.2033) (36.8629, -19.627) knots 0 0 0 1 2 2 2
  spline S101 degree 2 poles (36.8629, -19.627) (36.2042, -18.9375) (35.4632, -16.6218) (35.4632, -14.934) knots 0 0 0 1 2 2 2
  spline S102 degree 2 poles (35.4632, -14.934) (35.4632, -13.277) (36.1425, -10.6114) (36.8526, -9.6234) knots 0 0 0 1 2 2 2
  spline S103 degree 2 poles (36.8526, -9.6234) (37.5422, -8.656) (39.724, -7.5754) (41.1546, -7.5754) knots 0 0 0 1 2 2 2
  spline S104 degree 2 poles (41.1546, -7.5754) (41.5765, -7.5754) (42.3175, -7.6577) (42.5954, -7.7503) knots 0 0 0 1 2 2 2
  line L93 (42.5954, -7.7503) -> (42.5954, -9.3867)
  line L94 (42.5954, -9.3867) -> (42.5234, -9.3867)
  spline S105 degree 2 poles (42.5234, -9.3867) (42.2867, -9.2632) (41.4222, -9.0471) (40.9282, -9.0471) knots 0 0 0 1 2 2 2
  spline S106 degree 2 poles (40.9282, -9.0471) (39.3432, -9.0471) (37.3981, -11.1878) (37.2128, -13.2873) knots 0 0 0 1 2 2 2
  spline S107 degree 2 poles (37.2128, -13.2873) (37.82, -12.8653) (39.0962, -12.4022) (39.8578, -12.4022) knots 0 0 0 1 2 2 2
  spline S108 degree 2 poles (39.8578, -12.4022) (40.5988, -12.4022) (41.7103, -12.7007) (42.3175, -13.1535) knots 0 0 0 1 2 2 2
  spline S109 degree 2 poles (42.3175, -13.1535) (43.0174, -13.6784) (43.6966, -15.3045) (43.6966, -16.3954) knots 0 0 0 1 2 2 2
  spline S110 degree 2 poles (41.9676, -16.4674) (41.9676, -15.6853) (41.5559, -14.6252) (41.1031, -14.2547) knots 0 0 0 1 2 2 2
  spline S111 degree 2 poles (41.1031, -14.2547) (40.7635, -13.9871) (39.9196, -13.8122) (39.477, -13.8122) knots 0 0 0 1 2 2 2
  spline S112 degree 2 poles (39.477, -13.8122) (38.8801, -13.8122) (37.7583, -14.1724) (37.2128, -14.512) knots 0 0 0 1 2 2 2
  spline S113 degree 2 poles (37.2128, -14.512) (37.2025, -14.6973) (37.182, -15.0472) (37.182, -15.3148) knots 0 0 0 1 2 2 2
  spline S114 degree 2 poles (37.182, -15.3148) (37.182, -16.6321) (37.6965, -18.2479) (38.0876, -18.6699) knots 0 0 0 1 2 2 2
  spline S115 degree 2 poles (38.0876, -18.6699) (38.4478, -19.0712) (39.23, -19.3903) (39.6726, -19.3903) knots 0 0 0 1 2 2 2
  spline S116 degree 2 poles (39.6726, -19.3903) (40.7017, -19.3903) (41.9676, -17.9289) (41.9676, -16.4674) knots 0 0 0 1 2 2 2
  point P0 (0, 0)
  constraints: 2 other
emboss "Emboss1" sketch "Sketch14" operation cut depth 1.016 direction (0, 1, 0)
sketch "Sketch15" plane through (0, 0, 0) normal (0, -1, 0) x (1, 0, 0)
  point P0 (0, 0)
body "Solid1"
